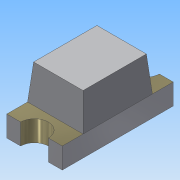
# Autodesk Inventor part: HSMG-C190 LED
Saved by Autodesk Inventor 2016 (Build 200138000, 138)
## iProperties
Created: 2019-08-19
Part Number: HSMG-C190 LED
Material: Generic
Document SubType Name: Modeling
Designer: Orest
Mass: 0.000708128 g
Surface Area: 0.0545803 cm^2
Volume: 0.000708128 cm^3
Density: 1 g/cm^3
Appearance: White
Author: Orest
Autodesk Inventor part; units mm, degrees
ref_plane "YZ Plane" through (0, 0, 0) normal (1, 0, 0) x (0, 1, 0)
ref_plane "XZ Plane" through (0, 0, 0) normal (0, 1, 0) x (-1, 0, 0)
ref_plane "XY Plane" through (0, 0, 0) normal (0, 0, 1) x (1, 0, 0)
sketch "Sketch10" plane through (0, 0, 0) normal (0, 1, 0) x (-1, 0, 0)
  line L0 (0.8, -0.4) -> (-0.8, -0.4)
  line L1 (-0.8, 0.4) -> (0.8, 0.4)
  arc A0 (0.8, 0.2) -> (0.8, -0.2) centre (0.8, 0) ccw
  arc A1 (-0.8, -0.2) -> (-0.8, 0.2) centre (-0.8, 0) ccw
  line L2 (0.8, 0.4) -> (0.8, 0.2)
  line L3 (0.8, -0.2) -> (0.8, -0.4)
  line L4 (-0.8, -0.4) -> (-0.8, -0.2)
  line L5 (-0.8, 0.2) -> (-0.8, 0.4)
  point P0 (0, 0)
  point P1 (0, -0.4)
  dimension "d7" = 1.6
  dimension "d8" = 0.8
  dimension "d9" = 0.2
  constraints: 12 end point, 5 parallel, 4 line through centre, 4 point on circle, 2 centre point, 2 collinear, 2 perpendicular, 1 coincident, 1 equal radius, 1 horizontal, 1 horizontal alignment, 1 midpoint, 1 vertical alignment
  measures "d7" distance of L0.start L0.end
  measures "d8" distance between parallel lines of L1 L0
  measures "d9" radius of A0
extrude "Extrusion4" add sketch "Sketch10" along normal blind 0.3
sketch "Sketch11" plane through (0, 0.3, 0) normal (0, 1, 0) x (1, 0, 0)
  line L0 (0.8, 0.4) -> (-0.8, 0.4) construction
  line L1 (-0.8, 0.4) -> (-0.8, 0.2) projected
  arc A0 (-0.8, -0.2) -> (-0.8, 0.2) centre (-0.8, 0) ccw projected
  line L2 (-0.8, -0.2) -> (-0.8, -0.4) projected
  line L3 (-0.8, -0.4) -> (0.8, -0.4) construction
  line L4 (0.8, -0.4) -> (0.8, -0.2) construction
  arc A1 (0.8, 0.2) -> (0.8, -0.2) centre (0.8, 0) ccw construction
  line L5 (0.8, 0.2) -> (0.8, 0.4) construction
  line L6 (-0.5, 0.4) -> (0.5, 0.4)
  line L7 (0.5, 0.4) -> (0.5, -0.4)
  line L8 (0.5, -0.4) -> (-0.5, -0.4)
  line L9 (-0.5, -0.4) -> (-0.5, 0.4)
  circle A2 centre (0, 0) radius 0.15
  circle A3 centre (0.65, 0.3) radius 0.05
  point P0 (0, 0.4)
  point P1 (0, -0.4)
  point P2 (0.5, 0)
  dimension "d12" = 1
  dimension "d13" = 0.8
  dimension "d16" = 0.3
  dimension "d20" = 0.15
  dimension "d21" = 0.1
  dimension "d22" = 0.1
  constraints: 8 end point, 4 midpoint, 2 centre point, 2 parallel, 1 collinear, 1 horizontal, 1 horizontal alignment, 1 perpendicular, 1 vertical alignment
  measures "d12" distance of L6.start L6.end
  measures "d13" distance of L8.end L6.start
  measures "d16" diameter of A2
  measures "d20" distance from line of L5 A3.centre
  measures "d21" distance from line of L0 A3.centre
  measures "d22" diameter of A3
extrude "Extrusion6" add sketch "Sketch11" along normal blind 0.1 contours A2
extrude "Extrusion5" add sketch "Sketch11" along normal blind 0.5 draft -5 contours L6 L7 L8 L9 | A2
extrude "Extrusion7" cut sketch "Sketch11" against normal blind 0.01 contours A3
body "Solid4"
